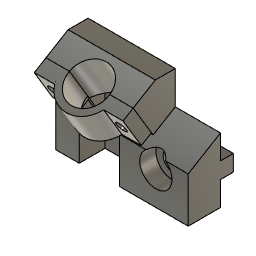
z_wire_up v3 (Autodesk Fusion 360 design; units mm, degrees)
Autodesk Fusion 360 part; units mm, degrees
note: some values were not read from the file. Set by a fixed rule: which sketch regions a step uses.
sketch "Sketch1" plane through (0, 0, 0) normal (0, 1, 0) x (1, 0, 0)
  circle A0 centre (0, 0) radius 2.75
  line L0 (10, -10) -> (-10, -10)
  line L1 (-10, -10) -> (-10, 10)
  line L2 (-10, 10) -> (10, 10)
  line L3 (10, 10) -> (10, -10)
  line L4 (10, -10) -> (-10, 10) construction
  line L5 (-10, -10) -> (10, 10) construction
  line L6 (-25, -2.5) -> (-21, -2.5)
  line L7 (-21, -2.5) -> (-21, 2.5)
  line L8 (-21, 2.5) -> (-25, 2.5)
  line L9 (-25, 2.5) -> (-25, -2.5)
  line L10 (6, 2.5) -> (6, -2.5)
  line L11 (6, -2.5) -> (10, -2.5)
  line L12 (10, 2.5) -> (6, 2.5)
  line L13 (10, -2.5) -> (10, 2.5)
  line L14 (-10, -10) -> (-25, -10)
  line L15 (-25, -10) -> (-25, 10)
  line L16 (-25, 10) -> (-10, 10)
  line L17 (-10, 10) -> (-10, -10)
  circle A1 centre (0, 0) radius 5
  line L18 (-25, -10) -> (-5, -10)
  line L19 (-5, -10) -> (-5, 10)
  line L20 (-5, 10) -> (-25, 10)
  line L21 (-25, 10) -> (-25, -10)
  line L22 (-25, -10) -> (-5, -10)
  line L23 (-5, -10) -> (-5, -20)
  line L24 (-5, -20) -> (-25, -20)
  line L25 (-25, -20) -> (-25, -10)
  line L26 (-25, 10) -> (-5, 10)
  line L27 (-5, 10) -> (-5, 15.5067)
  line L28 (-5, 15.5067) -> (-25, 15.5067)
  line L29 (-25, 15.5067) -> (-25, 10)
  dimension "d1" = 5.5
  dimension "d2" = 20
  dimension "d3" = 20
  dimension "d4" = 4
  dimension "d5" = 5
  dimension "d6" = 4
  dimension "d7" = 5
  dimension "d8" = 10
  dimension "d15" = 20
  dimension "d16" = 20
  constraint coincident A0.centre A1.centre
  constraint horizontal L0
  constraint perpendicular L0 L1
  constraint parallel L0 L2
  constraint parallel L1 L3
  constraint coincident L4 A0.centre
  constraint coincident L5 A0.centre
  constraint horizontal L6
  constraint vertical L7
  constraint horizontal L8
  constraint vertical L9
  constraint horizontal L11
  constraint vertical L13
  constraint horizontal L12
  constraint vertical L10
  constraint horizontal L14
  constraint vertical L15
  constraint horizontal L16
  constraint vertical L17
  constraint horizontal L18
  constraint vertical L19
  constraint horizontal L20
  constraint vertical L21
  constraint horizontal L22
  constraint vertical L23
  constraint horizontal L24
  constraint vertical L25
  constraint horizontal L26
  constraint vertical L27
  constraint horizontal L28
  constraint vertical L29
  measures "d1" diameter of A0
  measures "d2" distance of L1.end L2.end
  measures "d3" distance of L0.end L1.end
  measures "d4" distance of L6.start L6.end
  measures "d5" distance of L6.start L8.end
  measures "d6" distance of L10.end L11.end
  measures "d7" distance of L10.start L10.end
  measures "d8" diameter of A1
  measures "d15" distance of L14.end L18.end
  measures "d16" distance of L14.end L15.end
extrude "Extrude1" add sketch "Sketch1" along normal blind 14 contours L3 L10 L11 L12 L13 | L6 L7 L8 L9 L15 L21 makes body 1 at (-25, 4.6667, -0.8333) makes body 2 at (6, 4.6667, -0.8333)
extrude "Extrude2" add sketch "Sketch1" along normal blind 10 contours A1 | L0 L2 L3 L10 L11 L12 L19 | L0 L1 L2 L17 L18 L19 L20 L22 L26 | L1 L6 L7 L8 L14 L15 L16 L17 L18 L20 L21 L22 L26 bodies 1 2
extrude "Extrude3" cut sketch "Sketch1" along normal blind 5 contours A1 bodies 1
sketch "Sketch2" plane through (-25, 0, 0) normal (-1, 0, 0) x (0, -1, 0)
  line L0 (0, -10) -> (0, 10)
  line L1 (0, 10) -> (-10, 10)
  line L2 (-10, 10) -> (-10, 2.5)
  line L3 (-10, 2.5) -> (-14, 2.5)
  line L4 (-14, 2.5) -> (-14, -2.5)
  line L5 (-14, -2.5) -> (-10, -2.5)
  line L6 (-10, -2.5) -> (-10, -10)
  line L7 (-10, -10) -> (0, -10)
  line L8 (-10, 10) -> (0, 4)
  line L9 (0, 10) -> (0, 4)
  line L10 (0, 10) -> (-10, 10)
  constraint coincident L1.end L2.start
  constraint coincident L0 L8.end
  constraint coincident L0.end L1.start
  constraint perpendicular L1 L9
extrude "Extrude4" cut sketch "Sketch2" against normal blind 45 contours L0 L1 L8 L9 L10 bodies 1
sketch "Sketch3" plane through (0, -1.7647, 2.9412) normal (0, -0.514496, 0.857493) x (1, 0, 0)
  line L0 (-25, 13.7199) -> (-25, 2.058)
  line L1 (3, 2.058) -> (10, 2.058)
  line L2 (10, 13.7199) -> (-25, 13.7199)
  circle A0 centre (-17.5, 5.5) radius 6.25
  circle A1 centre (-17.5, 5.5) radius 8.2333
  ellipse E0 centre (0, -5.7166) end of major axis (0, -15.4349) minor radius 5 (3, 2.058) -> (-3, 2.058) ccw
  line L3 (10, 2.058) -> (10, 13.7199)
  line L4 (-25, 2.058) -> (-3, 2.058)
  line L5 (-4, 9.5) -> (-31, 9.5)
  line L6 (-31, 9.5) -> (-31, 1.5)
  line L7 (-31, 1.5) -> (-4, 1.5)
  line L8 (-4, 1.5) -> (-4, 9.5)
  line L9 (-4, 9.5) -> (-31, 1.5) construction
  line L10 (-31, 9.5) -> (-4, 1.5) construction
  line L11 (-25, 13.7199) -> (-31, 13.7199)
  line L12 (-31, 13.7199) -> (-31, 9.5)
  line L13 (-31, 1.5) -> (-31, -3)
  line L14 (-17.5, -2.7333) -> (-31, -2.7333)
  line L15 (-4, 9.5) -> (-4, 10)
  line L16 (-4, 10) -> (-4, 13.7199)
  line L17 (-4, 13.7199) -> (-25, 13.7199)
  line L18 (-4, 1.5) -> (-4, -2.7333)
  line L19 (-4, -2.7333) -> (-17.5, -2.7333)
  point P0 (-17.5, 5.5)
  dimension "d19" = 12.5
  dimension "d20" = 27
  dimension "d21" = 8
  constraint concentric A0 A1
  constraint horizontal L5
  constraint perpendicular L5 L6
  constraint parallel L5 L7
  constraint parallel L6 L8
  constraint coincident L9 P0
  constraint coincident L10 P0
  constraint coincident P0 A0.centre
  constraint coincident L0.start L2.end
  constraint perpendicular L6 L11
  constraint perpendicular L5 L12
  constraint perpendicular L7 L13
  constraint coincident A1 L14.start
  constraint coincident L13 L14.end
  constraint tangent A1 L14
  constraint perpendicular L13 L14
  constraint coincident L2 L16.end
  constraint perpendicular L2 L16
  constraint perpendicular L14 L18
  constraint tangent A1 L19
  measures "d19" diameter of A0
  measures "d20" distance of L6.end L7.end
  measures "d21" distance of L5.end L6.end
extrude "Extrude5" add sketch "Sketch3" along normal blind 12 separate body contours L0 L2 A1 L5 L17 | L0 L5 L11 L12 | L0 A1 L5 | L0 A1 L4 L5 L6 L7 | L2 A0 A1 L5 L17 | L0 A0 A1 L4 L5 | L0 A1 | L2 A1 L5 L15 L16 L17 | A1 L4 L5 L8 | A0 A1 L4 L5 | A0 A1 L4 L7 | A0 A1 L7 | A0 A1 L4 L7 makes body 3
extrude "Extrude6" add 1 faces at (-25, 6.6667, 5.5) along direction (-1, 0, 0) blind 6 on bodies 1 bodies 1
extrude "Extrude7" cut 1 faces at (-21, 11.3333, 0.8333) along direction (-1, 0, 0) blind 5 on bodies 1 bodies 1
extrude "Extrude8" cut sketch "Sketch3" against normal blind 27 contours A0 L4 L5 | A0 L5 | A0 L4 L7 | A0 L7 bodies 1
ref_plane "WorkPlane1" through (-17.5, 0.0531, 11.029) normal (0, 0.857493, 0.514496) x (-1, 0, 0)
split "Split1" by plane through (-17.5, 0.0531, 11.029) normal (0, 0.857493, 0.514496) bodies 3 makes body 4 at (-26.393, 1.0164, 18.6041)
extrude "Extrude9" cut 1 faces at (-29, 0.9001, 4.5401) along direction (0, -0.514496, 0.857493) blind 1 on bodies 3 bodies 3
sketch "Sketch4" plane through (-17.5, 1.0821, 9.314) normal (0, 0.857493, 0.514496) x (-1, 0, 0)
  line L0 (-13.5, -3) -> (-13.5, 8) construction
  line L1 (-7.4793, -3) -> (-13.5, -3) construction
  line L2 (13.5, -3) -> (7.1964, -3) construction
  line L3 (13.5, -3) -> (13.5, 8) construction
  line L4 (13.5, 8) -> (7.1964, -3) construction
  line L5 (-7.4793, -3) -> (-8.3257, -0.4851) construction
  line L6 (-8.3257, -0.4851) -> (-13.5, 8) construction
  circle A0 centre (10.3482, 2.5) radius 1.4
  circle A1 centre (10.3482, 2.5) radius 1.7
  circle A2 centre (-10.1518, 2.5) radius 1.7
  circle A3 centre (-10.1518, 2.5) radius 1.4
  dimension "d35" = 2.8
  dimension "d36" = 3.4
  dimension "d37" = 2.8
  dimension "d38" = 3.4
  constraint coincident L3.end L4.start
  constraint coincident L2.end L4.end
  constraint coincident L1.start L5.start
  constraint coincident L0.end L6.end
  constraint midpoint L4 A0.centre
  constraint concentric A0 A1
  constraint concentric A2 A3
  measures "d35" diameter of A0
  measures "d36" diameter of A1
  measures "d37" diameter of A3
  measures "d38" diameter of A2
extrude "Extrude10" cut sketch "Sketch4" against normal blind 7.5 contours A0 | A1 | A2 | A3 bodies 3
extrude "Extrude11" cut sketch "Sketch4" along normal blind 18 contours A0 | A3 bodies 4
sketch "Sketch5" plane through (-31, 0, 0) normal (-1, 0, 0) x (0, -1, 0)
  line L0 (0, 4) -> (-10, 10)
  line L1 (-10, 10) -> (-10, 2.5)
  line L2 (-10, 2.5) -> (-14, 2.5)
  line L3 (-14, 2.5) -> (-14, -2.5)
  line L4 (-14, -2.5) -> (-10, -2.5)
  line L5 (-10, -2.5) -> (-10, -10)
  line L6 (-10, -10) -> (0, -10)
  line L7 (0, -10) -> (0, 4)
  line L8 (-10, 10) -> (-3.8261, 20.2899)
  line L9 (-3.8261, 20.2899) -> (-10, 20.2899)
  line L10 (-10, 20.2899) -> (-10, 10)
  constraint coincident L8.end L9.start
  constraint horizontal L9
  constraint coincident L0.end L1.start
extrude "Extrude12" add sketch "Sketch5" against normal blind 27 contours L8 L9 L10 bodies 4 1
sketch "Sketch6" plane through (0, 0, 0) normal (0, -1, 0) x (1, 0, 0)
  ellipse E0 centre (-17.5, 10.6901) end of major axis (-17.5, -1.4577) minor radius 6.25 (-22.7168, 4) -> (-12.2832, 4) ccw
  line L0 (-22.7168, 4) -> (-31, 4)
  line L1 (-31, 4) -> (-31, -10)
  line L2 (-31, -10) -> (10, -10)
  line L3 (10, -10) -> (10, 4)
  line L4 (10, 4) -> (3, 4)
  arc A0 (-3, 4) -> (3, 4) centre (0, 0) ccw
  line L5 (-3, 4) -> (-12.2832, 4)
  line L6 (-23.7461, 5.884) -> (-11.2539, 5.884)
  line L7 (-11.2539, 5.884) -> (-11.2539, -10)
  line L8 (-11.2539, -10) -> (-23.7461, -10)
  line L9 (-23.7461, -10) -> (-23.7461, 5.884)
  point P0 (-23.7461, 5.884)
  point P1 (-11.2539, 5.884)
  constraint horizontal L6
  constraint vertical L7
  constraint horizontal L8
  constraint vertical L9
  constraint coincident L2 L7.end
  constraint coincident P0 L6.start
extrude "Extrude13" cut sketch "Sketch6" against normal blind 24 contours E0 L0 L5 L6 L7 L9 | E0 L0 L2 L5 L7 L8 L9 bodies 4
extrude "Extrude14" add sketch "Sketch6" along normal blind -10 and the other way blind 8 contours E0 L0 L5 L6 L7 L9 | E0 L0 L2 L5 L7 L8 L9 bodies 4
extrude "Extrude15" add 1 faces at (-19.3073, 8.6857, 5.884) along direction (0, 0, 1) blind 7 on bodies 4 bodies 4
named bodies: "z_wire_up_cap", "z_wire_up"
